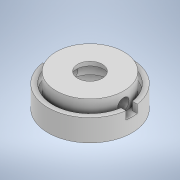
# Autodesk Inventor part: bottom seal v2
Saved by Autodesk Inventor 2022 (Build 260153000, 153)
## iProperties
Created: 2023-01-16
Part Number: bottom seal v2
Material: Generic
Document SubType Name: Modeling
Designer: ASUS
Density: 1 g/cm^3
Appearance: Default
Author: ASUS
Autodesk Inventor part; units mm, degrees
ref_plane "XZ Plane" through (0, 0, 0) normal (0, 1, 0) x (-1, 0, 0)
sketch "Sketch2" plane through (0, 0, 0) normal (0, 0, 1) x (1, 0, 0)
  line L0 (0, 0) -> (-20.875, 0)
  line L1 (-20.875, 0) -> (-20.875, -11.5)
  line L2 (-20.875, -11.5) -> (-22.875, -11.5)
  line L3 (-22.875, -11.5) -> (-22.875, -6.4943)
  line L4 (-22.875, -6.4943) -> (-25.875, -6.4943)
  line L5 (-25.875, -6.4943) -> (-25.875, -12.9943)
  line L6 (0, -3) -> (0, 0)
  line L7 (-25.875, -12.9943) -> (-25.875, -19.9943)
  line L8 (-25.875, -19.9943) -> (-14.1, -19.9943)
  line L9 (-14.1, 0) -> (-14.1, -19.9943) construction
  line L10 (-7.6, 0) -> (-7.6, -3) construction
  line L11 (-7.6, -3) -> (0, -3) construction
  line L12 (-7.6, 0) -> (-7.6, -10) construction
  line L13 (-8.349, -3) -> (-14.1, -3)
  line L14 (-14.1, -19.9943) -> (-14.1, -3)
  line L15 (-11.6, -3) -> (-11.6, -9.9943)
  line L16 (-11.6, -9.9943) -> (-14.1, -9.9943)
  line L17 (-7.6, 0) -> (-8.349, -3)
  dimension "d3" = 20.875
  dimension "d4" = 11.5
  dimension "d5" = 2
  dimension "d6" = 3
  dimension "d7" = 6.5
  dimension "d9" = 7
  dimension "d10" = 14.1
  dimension "d11" = 3
  dimension "d12" = 7.6
  dimension "d13" = 10
  dimension "d31" = 2.5
  dimension "d33" = 10
  constraints: 36 end point, 7 perpendicular, 6 vertical, 5 point on line, 2 horizontal
  measures "d3" distance of L0.start L0.end
  measures "d4" distance of L0.end L1.end
  measures "d5" distance of L1.end L2.end
  measures "d6" distance of L3.end L4.end
  measures "d7" distance of L4.end L5.end
  measures "d9" distance of L5.end L7.end
  measures "d10" distance between parallel lines of L6 L9
  measures "d11" distance of L10.start L10.end
  measures "d12" distance of L6.start L10.end
  measures "d13" distance of L10.start L12.end
  measures "d31" distance of L15.end L16.end
  measures "d33" distance from line of L8.end L16
revolve "Revolution1" add sketch "Sketch2" angle 360 about axis through (0, -3, 0) along (0, 1, 0)
sketch "Sketch3" plane through (0, 0, 0) normal (1, 0, 0) x (0, 1, 0)
  line L0 (0, -7.6) -> (0, 7.6) projected
  circle A0 centre (-7.05, 0) radius 3.5
  point P0 (0, 0)
  dimension "d16" = 7.05
  dimension "d17" = 0
  dimension "d20" = 7
  constraints: 1 centre point, 1 coincident
  measures "d16" distance from line of L0 point (-7.05, 0)
  measures "d17" vertical distance of point (0, 0) point (-7.05, 0)
  measures "d20" diameter of A0
extrude "Extrusion1" cut sketch "Sketch3" along normal through all both and the other way through all
ref_plane "Work Plane1" through (-28, 0, 0) normal (1, 0, 0) x (0, 1, 0)
sketch "Sketch4" plane through (-28, 0, 0) normal (1, 0, 0) x (0, 1, 0)
  line L0 (-11.5, -20.875) -> (-11.5, 20.875) projected
  line L1 (-6.4943, -3.4556) -> (-11.5, -3.4556)
  line L2 (-11.5, -3.4556) -> (-11.5, 3.5444)
  line L3 (-11.5, 3.5444) -> (-6.4943, 3.5444)
  line L4 (-6.4943, 3.5444) -> (-6.4943, -3.4556)
  point P0 (0, 0)
  dimension "d24" = 7
  constraints: 8 end point, 2 parallel, 1 horizontal, 1 perpendicular, 1 point on line
  measures "d24" distance of L3.end L1.start
extrude "Extrusion2" cut sketch "Sketch4" along normal up to surface
ref_plane "Work Plane2" through (28, 0, 0) normal (1, 0, 0) x (0, 1, 0)
sketch "Sketch5" plane through (28, 0, 0) normal (1, 0, 0) x (0, 1, 0)
  line L0 (-11.5, -20.875) -> (-11.5, 20.875) projected
  line L1 (-6.4943, 3.4556) -> (-11.5, 3.4556)
  line L2 (-11.5, 3.4556) -> (-11.5, -3.5444)
  line L3 (-11.5, -3.5444) -> (-6.4943, -3.5444)
  line L4 (-6.4943, -3.5444) -> (-6.4943, 3.4556)
  point P0 (0, 0)
  dimension "d28" = 7
  constraints: 8 end point, 2 parallel, 1 horizontal, 1 perpendicular, 1 point on line
  measures "d28" distance of L3.end L1.start
extrude "Extrusion3" cut sketch "Sketch5" against normal up to surface
body "Solid1"
